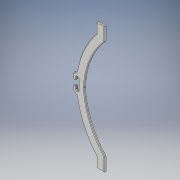
# Autodesk Inventor part: Baseplate_aussen
Saved by Autodesk Inventor 2018 (Build 220112000, 112)
## iProperties
Created: 2020-01-15
Part Number: Baseplate_aussen
Material: Generisch
Document SubType Name: Modeling
Designer: maxse
Density: 1 g/cm^3
Appearance: Vorgabe
Author: maxse
Autodesk Inventor part; units mm, degrees
ref_plane "YZ Plane" through (0, 0, 0) normal (1, 0, 0) x (0, 1, 0)
ref_plane "XZ Plane" through (0, 0, 0) normal (0, 1, 0) x (-1, 0, 0)
ref_plane "XY Plane" through (0, 0, 0) normal (0, 0, 1) x (1, 0, 0)
sketch "Skizze1" plane through (0, 0, 0) normal (0, 1, 0) x (-1, 0, 0)
  arc A0 (39, 0) -> (0, 95) centre (-110.879, -6.024) ccw
  line L0 (0, 95) -> (0, 120)
  line L1 (0, 120) -> (15, 120)
  line L2 (15, 120) -> (15, 100.6336)
  arc A1 (54, 0) -> (15, 100.6336) centre (-110.879, -6.024) ccw
  line L3 (39, 0) -> (54, 0)
  line L4 (0, 0) -> (39, 0)
  line L5 (59, 0) -> (59, 15)
  line L6 (59, 15) -> (52.765, 15)
  line L7 (59, 0) -> (54, 0)
  dimension "d0" = 25
  dimension "d2" = 15
  dimension "d4" = 54
  dimension "d5" = 0
  dimension "d6" = 120
  dimension "d7" = 150
  dimension "d9" = 5
  dimension "d10" = 15
  dimension "d11" = 15
  constraints: 16 end point, 6 point on circle, 3 perpendicular, 2 centre point, 2 horizontal, 2 vertical, 1 collinear, 1 concentric
  measures "d0" distance of L0.start L0.end
  measures "d2" distance of L0.end L1.end
  measures "d4" distance of L3.end L4.start
  measures "d5" distance from line of L4.start L0
  measures "d6" distance from line of L4.start L1
  measures "d7" radius of A0
  measures "d9" distance of L3.end L5.start
  measures "d10" distance of L3.end L3.start
  measures "d11" distance of L5.start L5.end
extrude "Extrusion1" add sketch "Skizze1" along normal blind 4
mirror "Spiegeln1" about plane through (-54, 0, 0) normal (0, 0, -1) of "Extrusion1"
sketch "Skizze2" plane through (0, 0, 0) normal (0, -1, 0) x (1, 0, 0)
  line L0 (-59, 15) -> (-59, -15) projected
  line L1 (-59, -5) -> (-54, -5)
  line L2 (-54, -5) -> (-54, -9.5)
  line L3 (-59, 5) -> (-54, 5)
  line L4 (-54, 5) -> (-54, 9.5)
  line L5 (-49, -9.5) -> (-49, 9.5)
  arc A0 (-49, 9.5) -> (-54, 9.5) centre (-51.5, 9.5) ccw
  arc A1 (-54, -9.5) -> (-49, -9.5) centre (-51.5, -9.5) ccw
  point P0 (0, 0)
  dimension "d15" = 10
  dimension "d16" = 5
  dimension "d17" = 10
  dimension "d18" = 5
  dimension "d19" = 5
  dimension "d20" = 24
  dimension "d21" = 4.5
  constraints: 10 end point, 4 point on circle, 4 tangent, 2 centre point, 2 horizontal, 2 point on line, 2 vertical, 1 perpendicular
  measures "d15" distance between parallel lines of L5 L0
  measures "d16" distance between parallel lines of L5 L2
  measures "d17" distance between parallel lines of L3 L1
  measures "d18" distance of L3.start L3.end
  measures "d19" distance from line of point (0, 0) L3
  measures "d21" distance from line of L1 A1.centre
extrude "Extrusion2" cut sketch "Skizze2" against normal blind 4
fillet "Rundung1" radius 10 3 edges at (-52.765, 2, -15) (-52.765, 2, 15) (-39, 2, 0)
fillet "Rundung2" radius 1 46 edges at (-7.5, 4, -120) (0, 4, -107.5) (-15, 4, -110.3168) (-7.5, 0, -120) (0, 0, -107.5) (-15, 0, -110.3168) (-54.0935, 4, -17.8718) (-38.4134, 4, -64.2123) (-54.0935, 0, -17.8718) (-38.4134, 0, -64.2123) (-38.9913, 4, 0) (-27.8012, 4, 51.1406) (-27.8012, 4, -51.1406) (-38.9913, 0, 0) (-27.8012, 0, 51.1406) (-27.8012, 0, -51.1406) (-54.0935, 4, 17.8718) (-38.4134, 4, 64.2123) (-54.0935, 0, 17.8718) (-38.4134, 0, 64.2123) (-59, 4, 10) (-59, 0, 10) (-59, 0, -10) (-59, 4, -10) (-59, 2, -5) (-59, 2, 5) (-54, 2, 5) (-54, 2, -5) (-56.5, 4, -5) (-56.5, 4, 5) (-51.5, 4, 12) (-54, 4, 7.25) (-51.5, 4, -12) (-54, 4, -7.25) (-49, 4, 0) (-51.5, 0, -12) (-54, 0, -7.25) (-51.5, 0, 12) (-54, 0, 7.25) (-49, 0, 0) (-15, 4, 110.3168) (-15, 0, 110.3168) (-7.5, 4, 120) (-7.5, 0, 120) (0, 0, 107.5) (0, 4, 107.5)
